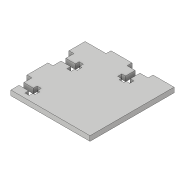
# Autodesk Inventor part: base
Saved by Autodesk Inventor 2017 (Build 210142000, 142)
## iProperties
Created: 2019-05-21
Part Number: base
Material: Generic
Document SubType Name: Modeling
Designer: markg
Density: 1 g/cm^3
Appearance: Default
Author: markg
Autodesk Inventor part; units mm, degrees
ref_plane "YZ Plane" through (0, 0, 0) normal (1, 0, 0) x (0, 1, 0)
ref_plane "XZ Plane" through (0, 0, 0) normal (0, 1, 0) x (-1, 0, 0)
ref_plane "XY Plane" through (0, 0, 0) normal (0, 0, 1) x (1, 0, 0)
sketch "Sketch1" plane through (0, 0, 0) normal (0, 1, 0) x (-1, 0, 0)
  line L0 (-25.4, 25.4) -> (25.4, 25.4)
  line L1 (25.4, 25.4) -> (25.4, -25.4)
  line L2 (25.4, -25.4) -> (-25.4, -25.4)
  line L3 (-25.4, -25.4) -> (-25.4, 25.4)
  line L4 (-25.4, 25.4) -> (25.4, -25.4) construction
  line L5 (25.4, 25.4) -> (-25.4, -25.4) construction
  point P0 (0, 0)
  dimension "d0" = 50.8
  dimension "d1" = 50.8
  constraints: 12 end point, 2 midpoint, 2 parallel, 1 horizontal, 1 perpendicular
  measures "d0" distance of L1.end L2.end
  measures "d1" distance of L0.end L1.end
extrude "Extrusion1" add sketch "Sketch1" along normal blind 2.9718
sketch "Sketch2" plane through (0, 2.9718, 0) normal (0, 1, 0) x (1, 0, 0)
  line L0 (-25.4, -25.4) -> (25.4, -25.4) projected
  line L1 (-25.4, -25.4) -> (-22.4282, -25.4)
  line L2 (-22.4282, -25.4) -> (-22.4282, -12.7)
  line L3 (-22.4282, -12.7) -> (-25.4, -12.7)
  line L4 (-25.4, -12.7) -> (-25.4, -25.4)
  line L5 (-25.4, 25.4) -> (-25.4, -25.4) projected
  line L6 (-25.4, 0) -> (-22.4282, 0)
  line L7 (-22.4282, 0) -> (-22.4282, 12.7)
  line L8 (-22.4282, 12.7) -> (-25.4, 12.7)
  line L9 (-25.4, 12.7) -> (-25.4, 0)
  line L10 (-25.4, 25.4) -> (-12.7, 25.4)
  line L11 (-12.7, 25.4) -> (-12.7, 22.4282)
  line L12 (-12.7, 22.4282) -> (-25.4, 22.4282)
  line L13 (-25.4, 22.4282) -> (-25.4, 25.4)
  line L14 (25.4, 25.4) -> (-25.4, 25.4) projected
  line L15 (0, 25.4) -> (12.7, 25.4)
  line L16 (12.7, 25.4) -> (12.7, 22.4282)
  line L17 (12.7, 22.4282) -> (0, 22.4282)
  line L18 (0, 22.4282) -> (0, 25.4)
  point P0 (0, 0)
  dimension "d4" = 2.9718
  dimension "d5" = 12.7
  dimension "d6" = 2.9718
  dimension "d7" = 12.7
  dimension "d8" = 12.7
  dimension "d9" = 2.9718
  dimension "d10" = 12.7
  dimension "d11" = 2.9718
  constraints: 32 end point, 8 parallel, 4 horizontal, 4 perpendicular, 2 midpoint
  measures "d4" distance of L3.end L2.end
  measures "d5" distance of L2.end L1.end
  measures "d6" distance of L8.end L7.end
  measures "d7" distance of L7.end L6.end
  measures "d8" distance of L11.end L12.end
  measures "d9" distance of L10.end L11.end
  measures "d10" distance of L16.end L17.end
  measures "d11" distance of L15.end L16.end
extrude "Extrusion2" cut sketch "Sketch2" against normal blind 2.9718
sketch "Sketch3" plane through (0, 0, 0) normal (0, -1, 0) x (1, 0, 0)
  line L0 (7.7851, -12.7) -> (4.9149, -12.7)
  line L1 (4.9149, -22.4282) -> (7.7851, -22.4282)
  line L2 (7.7851, -12.7) -> (4.9149, -22.4282) construction
  line L3 (4.9149, -12.7) -> (7.7851, -22.4282) construction
  line L4 (0, -22.4282) -> (12.7, -22.4282) projected
  line L5 (12.7, -22.4282) -> (12.7, -25.4) projected
  line L6 (2.6797, -14.0462) -> (2.6797, -16.5862)
  line L7 (10.0203, -16.5862) -> (10.0203, -14.0462)
  line L8 (10.0203, -14.0462) -> (2.6797, -16.5862) construction
  line L9 (2.6797, -14.0462) -> (10.0203, -16.5862) construction
  line L10 (2.6797, -16.5862) -> (4.9149, -16.5862)
  line L11 (4.9149, -12.7) -> (4.9149, -14.0462)
  line L12 (4.9149, -16.5862) -> (4.9149, -22.4282)
  line L13 (10.0203, -14.0462) -> (7.7851, -14.0462)
  line L14 (4.9149, -14.0462) -> (2.6797, -14.0462)
  line L15 (7.7851, -22.4282) -> (7.7851, -16.5862)
  line L16 (7.7851, -14.0462) -> (7.7851, -12.7)
  line L17 (7.7851, -16.5862) -> (10.0203, -16.5862)
  line L18 (-14.0462, -10.0203) -> (-16.5862, -10.0203)
  line L19 (-16.5862, -10.0203) -> (-16.5862, -7.7851)
  line L20 (-16.5862, -7.7851) -> (-22.4282, -7.7851)
  line L21 (-22.4282, -7.7851) -> (-22.4282, -4.9149)
  line L22 (-22.4282, -4.9149) -> (-16.5862, -4.9149)
  line L23 (-16.5862, -4.9149) -> (-16.5862, -2.6797)
  line L24 (-16.5862, -2.6797) -> (-14.0462, -2.6797)
  line L25 (-14.0462, -2.6797) -> (-14.0462, -4.9149)
  line L26 (-14.0462, -4.9149) -> (-12.7, -4.9149)
  line L27 (-12.7, -4.9149) -> (-12.7, -7.7851)
  line L28 (-12.7, -7.7851) -> (-14.0462, -7.7851)
  line L29 (-14.0462, -7.7851) -> (-14.0462, -10.0203)
  line L30 (-25.4, 0) -> (-22.4282, 0) projected
  line L31 (-22.4282, -12.7) -> (-22.4282, 0) projected
  line L32 (-14.0462, 17.6149) -> (-14.0462, 15.3797)
  line L33 (-12.7, 17.6149) -> (-14.0462, 17.6149)
  line L34 (-12.7, 20.4851) -> (-12.7, 17.6149)
  line L35 (-14.0462, 15.3797) -> (-16.5862, 15.3797)
  line L36 (-14.0462, 20.4851) -> (-12.7, 20.4851)
  line L37 (-14.0462, 22.7203) -> (-14.0462, 20.4851)
  line L38 (-16.5862, 22.7203) -> (-14.0462, 22.7203)
  line L39 (-16.5862, 15.3797) -> (-16.5862, 17.6149)
  line L40 (-16.5862, 20.4851) -> (-16.5862, 22.7203)
  line L41 (-22.4282, 20.4851) -> (-16.5862, 20.4851)
  line L42 (-16.5862, 17.6149) -> (-22.4282, 17.6149)
  line L43 (-22.4282, 17.6149) -> (-22.4282, 20.4851)
  point P0 (0, 0)
  point P1 (6.35, -17.5641)
  point P2 (6.35, -15.3162)
  dimension "d14" = 0
  dimension "d15" = 2.8702
  dimension "d16" = 6.35
  dimension "d17" = 9.7282
  dimension "d18" = 7.3406
  dimension "d19" = 0
  dimension "d20" = 2.54
  dimension "d22" = 5.842
  dimension "d23" = 2.2352
  dimension "d24" = 5.842
  dimension "d25" = 2.8702
  dimension "d26" = 1.3462
  dimension "d46" = 2.8702
  dimension "d47" = 5.842
  dimension "d48" = 2.2352
  dimension "d49" = 2.2352
  dimension "d50" = 1.3462
  dimension "d51" = 2.54
  dimension "d52" = 2.54
  dimension "d60" = 4.9149
  dimension "d61" = 0
  dimension "d64" = 25.4
  constraints: 80 end point, 12 point on line, 11 perpendicular, 10 parallel, 4 midpoint, 3 horizontal, 2 collinear, 1 vertical, 23 other
  measures "d14" distance between parallel lines of L4 L1
  measures "d15" distance of L0.start L0.end
  measures "d16" distance from line of L5 point (6.35, -17.564)
  measures "d17" distance of L1.end L0.start
  measures "d18" distance of L7.end L6.start
  measures "d19" horizontal distance of point (6.35, -17.564) point (6.35, -15.316)
  measures "d20" distance of L6.start L6.end
  measures "d22" distance of L1.end L15.end
  measures "d23" distance of L15.end L7.start
  measures "d24" distance of L10.end L1.start
  measures "d25" distance of L1.start L1.end
  measures "d26" distance of L13.end L0.start
  measures "d46" distance of L21.start L21.end
  measures "d47" distance of L21.end L23.start
  measures "d48" distance of L19.start L19.end
  measures "d49" distance of L23.start L23.end
  measures "d50" distance of L27.end L29.start
  measures "d51" distance of L23.end L24.end
  measures "d52" distance of L18.start L19.start
  measures "d60" distance between parallel lines of L30 L22
  measures "d61" distance between parallel lines of L31 L21
  measures "d64" distance of L18.start L32.end
extrude "Extrusion4" cut sketch "Sketch3" against normal blind 25.4
body "Solid1"
